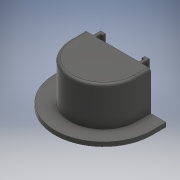
# Autodesk Inventor part: Prise
Saved by Autodesk Inventor 2017 (Build 210142000, 142)
## iProperties
Company: FABLAB Frenchmakers
Part Number: Prise
Material: Plastique ABS
Document SubType Name: Modeling
Designer: FABLAB Frenchmakers
Density: 1.06 g/cm^3
Appearance: Lisse - Blanc(1)
Mass: 44.018 g
Surface Area: 124.311 cm^2
Volume: 41.5264 cm^3
Project: 1400-PopCorn Machine
Stock Number: 1400-01-08
Author: Adrien MARY
Autodesk Inventor part; units mm, degrees
ref_plane "YZ Plane" through (0, 0, 0) normal (1, 0, 0) x (0, 1, 0)
ref_plane "XZ Plane" through (0, 0, 0) normal (0, 1, 0) x (-1, 0, 0)
ref_plane "XY Plane" through (0, 0, 0) normal (0, 0, 1) x (1, 0, 0)
sketch "Esquisse1" plane through (0, 0, 0) normal (0, 0, 1) x (1, 0, 0)
  arc A0 (-35, 0) -> (35, 0) centre (0, 0) ccw
  line L0 (-35, 0) -> (-35, 10)
  line L1 (-35, 10) -> (35, 10)
  line L2 (35, 10) -> (35, 0)
  dimension "d0" = 70
  dimension "d1" = 10
  constraints: 6 end point, 2 point on circle, 2 tangent, 2 vertical, 1 centre point, 1 coincident, 1 perpendicular
  measures "d0" diameter of A0
  measures "d1" distance from line of A0.centre L1
extrude "Extrusion1" add sketch "Esquisse1" along normal blind 3
sketch "Esquisse2" plane through (0, 0, 3) normal (0, 0, 1) x (1, 0, 0)
  arc A0 (-24, 0) -> (24, 0) centre (0, 0) ccw
  line L0 (35, 10) -> (-35, 10) projected
  line L1 (-33.1295, -24) -> (42.942, -24) construction
  line L2 (-24, 0) -> (-24, 10)
  line L3 (24, 0) -> (24, 10)
  line L4 (-24, 10) -> (24, 10)
  dimension "d5" = 34
  constraints: 8 end point, 3 tangent, 2 point on circle, 2 point on line, 2 vertical, 1 centre point, 1 coincident, 1 collinear, 1 horizontal
  measures "d5" distance between parallel lines of L0 L1
extrude "Extrusion2" add sketch "Esquisse2" along normal blind 28
fillet "Congé1" radius 2 3 edges at (0, -24, 31) (-24, 5, 31) (24, 5, 31)
sketch "Esquisse3" plane through (0, 0, 31) normal (0, 0, 1) x (1, 0, 0)
  line L0 (-17.5, 10) -> (-17.5, 15.5)
  line L1 (-17.5, 15.5) -> (-14.2, 15.5)
  line L2 (-14.2, 15.5) -> (-14.2, 13.5)
  line L3 (-14.2, 13.5) -> (-15.5, 13.5)
  line L4 (-15.5, 13.5) -> (-15.5, 10)
  line L5 (-15.5, 10) -> (-17.5, 10)
  line L6 (22, 10) -> (-22, 10) projected
  line L7 (0, -45.6195) -> (0, 28.7169) construction
  line L8 (17.5, 10) -> (17.5, 15.5)
  line L9 (17.5, 15.5) -> (14.2, 15.5)
  line L10 (14.2, 15.5) -> (14.2, 13.5)
  line L11 (14.2, 13.5) -> (15.5, 13.5)
  line L12 (15.5, 13.5) -> (15.5, 10)
  line L13 (15.5, 10) -> (17.5, 10)
  point P0 (0, 0)
  dimension "d9" = 35
  dimension "d10" = 31
  dimension "d11" = 2
  dimension "d12" = 5.5
  dimension "d13" = 3.3
  constraints: 24 end point, 6 symmetric about line, 5 perpendicular, 1 collinear, 1 vertical
  measures "d9" diameter of L0 L7
  measures "d10" diameter of L4 L7
  measures "d11" distance between parallel lines of L1 L3
  measures "d12" distance between parallel lines of L5 L1
  measures "d13" distance between parallel lines of L0 L2
extrude "Extrusion3" add sketch "Esquisse3" against normal up to surface (31 mm away)
sketch "Esquisse4" plane through (-15.5, 10, 0) normal (0, 1, 0) x (1, 0, 0)
  line L0 (28, -8.5) -> (3, -8.5)
  line L1 (3, -8.5) -> (3, -25)
  line L2 (3, -25) -> (28, -25)
  line L3 (28, -25) -> (28, -8.5)
  line L4 (31, 0) -> (0, 0) projected
  line L5 (31, -31) -> (0, -31) projected
  point P0 (15.5, 0)
  point P1 (15.5, -8.5)
  point P2 (15.5, 0)
  dimension "d16" = 25
  dimension "d17" = 16.5
  dimension "d18" = 6
  constraints: 8 end point, 2 midpoint, 2 parallel, 1 horizontal, 1 perpendicular, 1 vertical alignment
  measures "d16" distance between parallel lines of L1 L3
  measures "d17" distance between parallel lines of L0 L2
  measures "d18" distance between parallel lines of L5 L2
extrude "Extrusion4" cut sketch "Esquisse4" against normal blind 16
chamfer "Chanfrein1" distance 4 angle 45 2 edges at (12.5, 2, 8.5) (-12.5, 2, 8.5)
fillet "Congé3" radius 4 2 edges at (-12.5, 2, 25) (12.5, 2, 25)
fillet "Congé3" radius 2 4 edges at (8.5, 2, 8.5) (12.5, 2, 12.5) (-8.5, 2, 8.5) (-12.5, 2, 12.5)
sketch "Esquisse5" plane through (-15.5, -6, 0) normal (0, 1, 0) x (1, 0, 0)
  line L0 (23.5, -18.5) -> (21.5, -18.5)
  line L1 (21.5, -18.5) -> (21.5, -22.5)
  line L2 (21.5, -22.5) -> (23.5, -22.5)
  line L3 (23.5, -22.5) -> (23.5, -18.5)
  line L4 (9.5, -18.5) -> (7.5, -18.5)
  line L5 (7.5, -18.5) -> (7.5, -22.5)
  line L6 (7.5, -22.5) -> (9.5, -22.5)
  line L7 (9.5, -22.5) -> (9.5, -18.5)
  line L8 (16.5, -11) -> (14.5, -11)
  line L9 (14.5, -11) -> (14.5, -15)
  line L10 (14.5, -15) -> (16.5, -15)
  line L11 (16.5, -15) -> (16.5, -11)
  line L12 (7.8284, -8.5) -> (23.1716, -8.5) projected
  line L13 (24, -25) -> (7, -25) projected
  point P0 (15.5, 0)
  point P1 (15.5, -11)
  dimension "d27" = 2
  dimension "d28" = 2
  dimension "d29" = 2
  dimension "d30" = 12
  dimension "d31" = 6
  dimension "d32" = 4
  dimension "d33" = 4
  dimension "d34" = 2.5
  dimension "d35" = 2.5
  constraints: 24 end point, 6 parallel, 3 horizontal, 3 perpendicular, 2 point on line, 1 midpoint, 1 vertical alignment
  measures "d27" distance between parallel lines of L3 L1
  measures "d28" distance between parallel lines of L9 L11
  measures "d29" distance between parallel lines of L5 L7
  measures "d30" distance between parallel lines of L7 L1
  measures "d31" distance from line of point (15.5, 0) L1
  measures "d32" distance between parallel lines of L2 L0
  measures "d33" distance between parallel lines of L8 L10
  measures "d34" distance between parallel lines of L12 L8
  measures "d35" distance between parallel lines of L13 L2
extrude "Extrusion5" add sketch "Esquisse5" along normal blind 15 separate body
chamfer "Chanfrein2" distance 1 angle 45 12 edges at (6, 9, 20.5) (7, 9, 22.5) (8, 9, 20.5) (7, 9, 18.5) (-1, 9, 13) (0, 9, 15) (1, 9, 13) (0, 9, 11) (-7, 9, 18.5) (-6, 9, 20.5) (-7, 9, 22.5) (-8, 9, 20.5)
equation "\"d28\" = d27"
equation "\"d29\" = d27"
equation "\"d31\" = 0.5 * d30"
equation "\"d33\" = d32"
equation "\"d35\" = d34"
equation "\"nombredor\" = 1.61803"
equation "\"pi\" = 3.141593"
